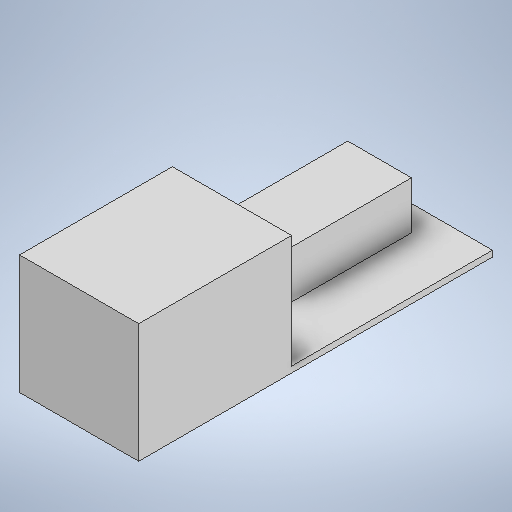
# Autodesk Inventor part: PCB Board
Saved by Autodesk Inventor 2025 (Build 290162000, 162)
## iProperties
Created: 2024-07-09
Part Number: PCB Board
Material: Generic
Document SubType Name: Modeling
Designer: track
Density: 1 g/cm^3
Appearance: Default
Author: track
Autodesk Inventor part; units mm, degrees
ref_plane "YZ Plane" through (0, 0, 0) normal (1, 0, 0) x (0, 1, 0)
ref_plane "XZ Plane" through (0, 0, 0) normal (0, 1, 0) x (-1, 0, 0)
ref_plane "XY Plane" through (0, 0, 0) normal (0, 0, 1) x (1, 0, 0)
sketch "Sketch1" plane through (0, 0, 0) normal (0, 1, 0) x (-1, 0, 0)
  line L0 (16.375, 48.6) -> (-16.375, 48.6)
  line L1 (-16.375, 48.6) -> (-16.375, -48.6)
  line L2 (-16.375, -48.6) -> (16.375, -48.6)
  line L3 (16.375, -48.6) -> (16.375, 48.6)
  line L4 (16.375, 48.6) -> (-16.375, -48.6) construction
  line L5 (-16.375, 48.6) -> (16.375, -48.6) construction
  point P0 (0, 0)
  dimension "d0" = 32.75
  dimension "d1" = 97.2
  constraints: 12 end point, 2 midpoint, 2 parallel, 1 horizontal, 1 perpendicular
  measures "d0" distance of L0.start L0.end
  measures "d1" distance of L0.end L1.end
extrude "Extrusion1" add sketch "Sketch1" along normal blind 1.65
sketch "Sketch2" plane through (0, 1.65, 0) normal (0, 1, 0) x (1, 0, 0)
  line L0 (-16.375, -48.6) -> (16.375, -48.6) projected
  line L1 (16.375, -48.6) -> (16.375, 48.6) projected
  line L2 (-16.375, -48.6) -> (16.375, -48.6)
  line L3 (16.375, -48.6) -> (16.375, -6.6)
  line L4 (16.375, -6.6) -> (-16.375, -6.6)
  line L5 (-16.375, -6.6) -> (-16.375, -48.6)
  point P0 (0, 0)
  dimension "d4" = 42
  constraints: 8 end point, 2 parallel, 1 horizontal, 1 perpendicular, 1 point on line
  measures "d4" distance of L4.end L0.start
extrude "Extrusion2" add sketch "Sketch2" along normal blind 31.1
sketch "Sketch3" plane through (0, 1.65, 0) normal (0, 1, 0) x (1, 0, 0)
  line L0 (-16.375, 48.6) -> (-16.375, -48.6) projected
  line L1 (-16.375, 41.6) -> (1.125, 41.6)
  line L2 (1.125, 41.6) -> (1.125, 1.1)
  line L3 (1.125, 1.1) -> (-16.375, 1.1)
  line L4 (-16.375, 1.1) -> (-16.375, 41.6)
  line L5 (16.375, 48.6) -> (-16.375, 48.6) projected
  point P0 (0, 0)
  dimension "d7" = 17.5
  dimension "d8" = 40.5
  dimension "d9" = 7
  constraints: 8 end point, 2 parallel, 1 horizontal, 1 perpendicular, 1 point on line
  measures "d7" distance of L1.start L1.end
  measures "d8" distance of L1.end L2.end
  measures "d9" distance between parallel lines of L5 L1
extrude "Extrusion3" add sketch "Sketch3" along normal blind 13.1
body "Solid1"
